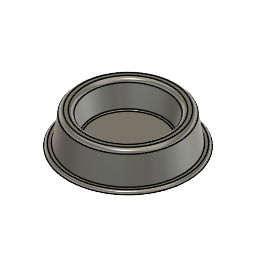
Day 11 Dog Bowl (Autodesk Fusion 360 design; units mm, degrees)
part number: 2026-07-14-23-25-55-717
part number: 2026-07-14-23-27-46-341
part number: 2026-07-14-23-28-48-822
Autodesk Fusion 360 part; units mm, degrees
sketch "Sketch1" plane through (0, 0, 0) normal (0, 0, 1) x (1, 0, 0) in component "Metal Bowl"
  line L0 (0, 0) -> (110, 0) construction
  line L1 (110, 0) -> (110, 2.5)
  line L2 (110, 2.5) -> (100, 2.5)
  line L3 (100, 2.5) -> (90.4494, 56.6644)
  line L4 (90.4494, 56.6644) -> (75.4494, 56.6644)
  line L5 (75.4494, 56.6644) -> (67.2212, 10)
  line L6 (0, 10) -> (67.2212, 10)
  dimension "d1" = 110
  dimension "d2" = 2.5
  dimension "d3" = 10
  dimension "d4" = 100
  dimension "d5" = 55
  dimension "d6" = 15
  dimension "d7" = 10
  dimension "d8" = 100
  constraint coincident L0.start origin
  constraint horizontal L0
  constraint perpendicular L0 L1
  constraint perpendicular L1 L2
  constraint parallel L0 L4
  constraint horizontal L6
  constraint vertical L0.start L6.start
  measures "d1" distance of L0.start L0.end
  measures "d2" distance of L0.end L1.end
  measures "d3" distance of L1.end L2.end
  measures "d4" angle of L2 L3
  measures "d5" distance of L2.end L3.end
  measures "d6" distance of L3.end L4.end
  measures "d7" distance of L0 L6
  measures "d8" angle of L5 L6
surface "Revolve1" add revolved angle 360 about axis through (0, 1.75, 0) along (0, 20.75, 0) path "Sketch1" along L1 L2 L3 L4 L5 L6 makes body 1 in component "Metal Bowl"
fillet "Fillet1" radius 5 2 edges at (-84.3284, 56.6644, -32.7079) (-70.3435, 56.6644, -27.2836) on bodies 1 in component "Metal Bowl"
fillet "Fillet2" radius 5 1 edges at (-62.6721, 10, -24.3082) on bodies 1 in component "Metal Bowl"
fillet "Fillet3" radius 2.5 2 edges at (-102.556, 2.5, -39.7777) (-93.2327, 2.5, -36.1615) on bodies 1 in component "Metal Bowl"
thicken "Thicken1" add thickness 2.5 surfaces 1 separate body makes body 2 in component "Metal Bowl"
sketch "Sketch1 (2)" plane through (0, 2.5, 0) normal (0, -1, 0) x (1, 0, 0) in component "Rubber grip"
  circle A0 centre (0, 0) radius 107.5
  circle A1 centre (0, 0) radius 102.0977
component "Metal Bowl" placed x (1, 0, 0) y (0, 1, 0) z (0, 0, 1) at (0, 0, 0)
component "Rubber grip" placed x (1, 0, 0) y (0, 1, 0) z (0, 0, 1) at (0, 0, 0)
hidden bodies 1
